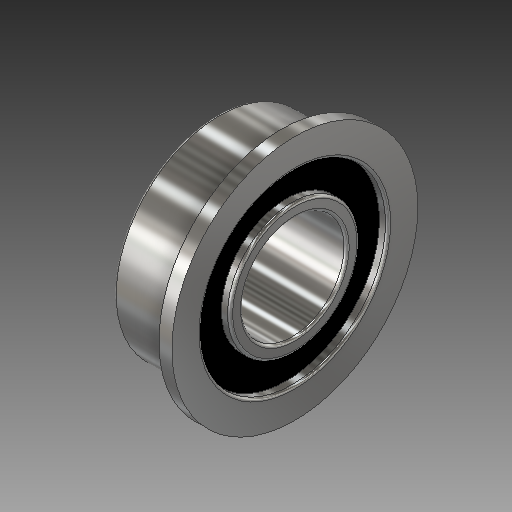
# Autodesk Inventor part: Подшипник 685
Saved by Autodesk Inventor 2018 (Build 220112000, 112)
## iProperties
Part Number: Подшипник 685
Material: Типовые
Document SubType Name: Modeling
Designer: sbnnl
Density: 1 g/cm^3
Appearance: Хром - полированный
Author: sbnnl
Autodesk Inventor part; units mm, degrees
ref_plane "YZ Plane" through (0, 0, 0) normal (1, 0, 0) x (0, 1, 0)
ref_plane "XZ Plane" through (0, 0, 0) normal (0, 1, 0) x (-1, 0, 0)
ref_plane "XY Plane" through (0, 0, 0) normal (0, 0, 1) x (1, 0, 0)
sketch "Эскиз1" plane through (0, 0, 0) normal (1, 0, 0) x (0, 1, 0)
  circle A0 centre (0, 0) radius 2
  circle A1 centre (0, 0) radius 4
  dimension "d0" = 4
  dimension "d1" = 8
  constraints: 2 centre point, 2 coincident
  measures "d0" diameter of A0
  measures "d1" diameter of A1
extrude "Выдавливание1" add sketch "Эскиз1" along normal blind 3
sketch "Эскиз2" plane through (3, 0, 0) normal (1, 0, 0) x (0, 0, -1)
  circle A0 centre (0, 0) radius 2.5
  circle A1 centre (0, 0) radius 3.6
  circle A2 centre (0, 0) radius 4 projected
  circle A3 centre (0, 0) radius 2 projected
  dimension "d4" = 5
  dimension "d5" = 7.2
  dimension "d15" = 8
  dimension "d16" = 4
  constraints: 2 centre point, 2 coincident
  measures "d4" diameter of A0
  measures "d5" diameter of A1
  measures "d15" diameter of A2
  measures "d16" diameter of A3
extrude "Выдавливание2" cut sketch "Эскиз2" against normal blind 0.3333 contours A1
sketch "Эскиз3" plane through (0, 0, 0) normal (-1, 0, 0) x (0, 0, 1)
  circle A0 centre (0, 0) radius 2.5 projected
  circle A1 centre (0, 0) radius 3.6 projected
  circle A2 centre (0, 0) radius 2.5
  circle A3 centre (0, 0) radius 3.6
  constraints: 2 centre point, 2 coincident, 2 concentric
extrude "Выдавливание3" cut sketch "Эскиз3" against normal blind 0.3333
fillet "Сопряжение1" radius 0.1 8 edges at (3, -4, 0) (3, 0, 3.6) (3, 0, 2.5) (3, -2, 0) (0, -4, 0) (0, 0, -3.6) (0, 0, -2.5) (0, -2, 0)
sketch "Эскиз6" plane through (3, 0, 0) normal (1, 0, 0) x (0, 0, -1)
  circle A0 centre (0, 0) radius 4.75
  circle A1 centre (0, 0) radius 3.9 projected
  dimension "d17" = 9.5
  constraints: 1 centre point, 1 coincident
  measures "d17" diameter of A0
extrude "Выдавливание6" add sketch "Эскиз6" against normal blind 0.5
equation "\"d4\" = 1.25 * d16"
equation "\"d5\" = 0.9 * d15"
equation "\"d6\" = 0.0833333 * d0"
equation "\"d8\" = 0.0833333 * d0"
